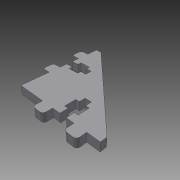
# Autodesk Inventor part: z_motor_brace
Saved by Autodesk Inventor 2014 (Build 180170000, 170)
## iProperties
Created: 2013-12-06
Part Number: z_motor_brace
Material: Generic
Document SubType Name: Modeling
Designer: buben
Density: 1 g/cm^3
Appearance: Default
Author: buben
Subject: Laser Cutted
Autodesk Inventor part; units mm, degrees
ref_plane "YZ Plane" through (0, 0, 0) normal (1, 0, 0) x (0, 1, 0)
ref_plane "XZ Plane" through (0, 0, 0) normal (0, 1, 0) x (-1, 0, 0)
ref_plane "XY Plane" through (0, 0, 0) normal (0, 0, 1) x (1, 0, 0)
sketch "Sketch1" plane through (0, 0, 0) normal (0, 0, 1) x (1, 0, 0)
  line L0 (0, 58) -> (0, 0)
  line L1 (0, 0) -> (58, 0)
  line L2 (58, 0) -> (58, 4)
  line L3 (58, 4) -> (4, 58)
  line L4 (4, 58) -> (0, 58)
  dimension "d0" = 58
  dimension "d1" = 4
  dimension "d2" = 4
  constraints: 10 end point, 3 perpendicular, 1 parallel, 1 vertical
  measures "d0" distance of L0.end L1.end
  measures "d1" distance of L1.end L2.end
  measures "d2" distance of L3.end L0.start
extrude "Extrusion1" add sketch "Sketch1" along normal blind 6
sketch "Sketch4" plane through (0, 0, 6) normal (0, 0, 1) x (1, 0, 0)
  line L0 (0, 58) -> (0, 0) projected
  line L1 (0, 0) -> (58, 0) projected
  line L2 (0, 19) -> (-4, 19)
  line L3 (-6, 21) -> (-6, 25)
  line L4 (-4, 27) -> (0, 27)
  line L5 (0, 27) -> (0, 19)
  line L6 (0, 42) -> (-4, 42)
  line L7 (-6, 44) -> (-6, 48)
  line L8 (-4, 50) -> (0, 50)
  line L9 (0, 50) -> (0, 42)
  line L10 (19, 0) -> (27, 0)
  line L11 (27, 0) -> (27, -4)
  line L12 (25, -6) -> (21, -6)
  line L13 (19, -4) -> (19, 0)
  line L14 (42, 0) -> (50, 0)
  line L15 (50, 0) -> (50, -4)
  line L16 (48, -6) -> (44, -6)
  line L17 (42, -4) -> (42, 0)
  arc A0 (-4, 50) -> (-6, 48) centre (-4, 48) ccw
  arc A1 (-6, 44) -> (-4, 42) centre (-4, 44) ccw
  arc A2 (-4, 27) -> (-6, 25) centre (-4, 25) ccw
  arc A3 (-6, 21) -> (-4, 19) centre (-4, 21) ccw
  arc A4 (19, -4) -> (21, -6) centre (21, -4) ccw
  arc A5 (25, -6) -> (27, -4) centre (25, -4) ccw
  arc A6 (42, -4) -> (44, -6) centre (44, -4) ccw
  arc A7 (48, -6) -> (50, -4) centre (48, -4) ccw
  dimension "d30" = 2
  dimension "d31" = 8
  dimension "d32" = 8
  dimension "d33" = 8
  dimension "d34" = 8
  dimension "d35" = 6
  dimension "d36" = 6
  dimension "d37" = 15
  dimension "d38" = 15
  dimension "d39" = 19
  dimension "d40" = 19
  constraints: 32 end point, 16 point on circle, 16 tangent, 8 centre point, 8 parallel, 7 equal radius, 4 horizontal, 4 perpendicular, 4 point on line, 2 collinear
  measures "d30" radius of A0
  measures "d31" distance between parallel lines of L6 L8
  measures "d32" distance between parallel lines of L2 L4
  measures "d33" distance between parallel lines of L11 L13
  measures "d34" distance between parallel lines of L15 L17
  measures "d35" distance between parallel lines of L7 L9
  measures "d36" distance between parallel lines of L1 L16
  measures "d37" distance between parallel lines of L17 L11
  measures "d38" distance between parallel lines of L4 L6
  measures "d39" distance from line of L0.end L13
  measures "d40" distance from line of L2 L0.end
extrude "Extrusion3" add sketch "Sketch4" against normal blind 6
sketch "Sketch5" plane through (0, 0, 6) normal (0, 0, 1) x (1, 0, 0)
  line L0 (0, 42) -> (0, 27) projected
  line L1 (0, 27) -> (-4, 27) projected
  line L2 (27, 0) -> (42, 0) projected
  line L3 (42, 0) -> (42, -4) projected
  line L4 (16.3, 36.75) -> (16.3, 32.25)
  line L5 (0, 32.25) -> (0, 36.75)
  line L6 (5, 39.25) -> (12.3, 39.25)
  line L7 (12.3, 29.75) -> (5, 29.75)
  line L8 (32.25, 16.3) -> (36.75, 16.3)
  line L9 (36.75, 0) -> (32.25, 0)
  line L10 (39.25, 12.3) -> (39.25, 5)
  line L11 (29.75, 5) -> (29.75, 12.3)
  line L12 (0, 36.75) -> (5, 36.75)
  line L13 (12.3, 36.75) -> (16.3, 36.75)
  line L14 (16.3, 32.25) -> (12.3, 32.25)
  line L15 (5, 32.25) -> (0, 32.25)
  line L16 (5, 29.75) -> (5, 32.25)
  line L17 (5, 36.75) -> (5, 39.25)
  line L18 (12.3, 39.25) -> (12.3, 36.75)
  line L19 (12.3, 32.25) -> (12.3, 29.75)
  line L20 (32.25, 0) -> (32.25, 5)
  line L21 (32.25, 12.3) -> (32.25, 16.3)
  line L22 (36.75, 16.3) -> (36.75, 12.3)
  line L23 (36.75, 5) -> (36.75, 0)
  line L24 (29.75, 12.3) -> (32.25, 12.3)
  line L25 (36.75, 12.3) -> (39.25, 12.3)
  line L26 (39.25, 5) -> (36.75, 5)
  line L27 (32.25, 5) -> (29.75, 5)
  point P0 (16.3, 34.5)
  point P1 (34.5, 16.3)
  dimension "d43" = 4.5
  dimension "d44" = 4.5
  dimension "d45" = 5
  dimension "d46" = 4
  dimension "d47" = 7.3
  dimension "d48" = 4
  dimension "d49" = 5
  dimension "d50" = 7.3
  dimension "d51" = 2.5
  dimension "d52" = 2.5
  dimension "d53" = 2.5
  dimension "d54" = 2.5
  dimension "d55" = 7.5
  dimension "d56" = 7.5
  constraints: 48 end point, 20 parallel, 10 collinear, 8 perpendicular, 6 horizontal, 2 midpoint
  measures "d43" distance of L8.start L8.end
  measures "d44" distance of L4.start L4.end
  measures "d45" distance of L5.end L12.end
  measures "d46" distance of L13.start L4.start
  measures "d47" distance of L6.start L6.end
  measures "d48" distance of L21.start L8.start
  measures "d49" distance of L9.end L20.end
  measures "d50" distance of L11.start L11.end
  measures "d51" distance of L12.end L6.start
  measures "d52" distance of L7.end L15.start
  measures "d53" distance of L20.end L11.start
  measures "d54" distance of L10.end L23.start
  measures "d55" distance from line of L1 point (16.3, 34.5)
  measures "d56" distance from line of L3 point (34.5, 16.3)
extrude "Extrusion4" cut sketch "Sketch5" against normal blind 6
body "Solid1"
